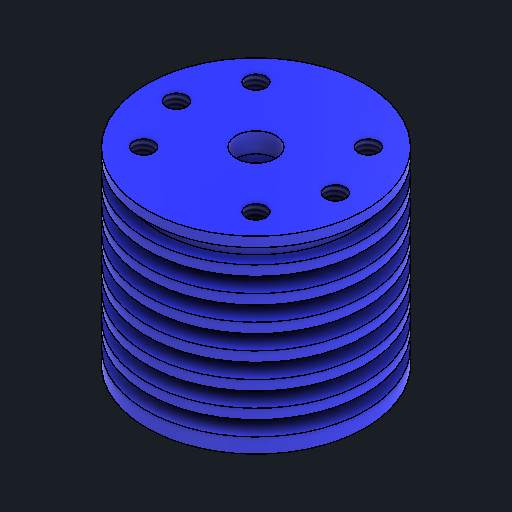
# Autodesk Inventor part: Radiator
Saved by Autodesk Inventor 2026.1 (Build 301233020, 233B)
## iProperties
Created: 2025-11-13
Part Number: Radiator
Material: Aluminum 6061
Document SubType Name: Modeling
Designer: JoshuaEah
Density: 2.7 g/cm^3
Appearance: Blue - Wall Paint - Glossy
Author: JoshuaEah
Autodesk Inventor part; units mm, degrees
ref_plane "YZ Plane" through (0, 0, 0) normal (1, 0, 0) x (0, 1, 0)
ref_plane "XZ Plane" through (0, 0, 0) normal (0, 1, 0) x (-1, 0, 0)
ref_plane "XY Plane" through (0, 0, 0) normal (0, 0, 1) x (1, 0, 0)
sketch "Sketch1" plane through (0, 0, 0) normal (0, 1, 0) x (-1, 0, 0)
  circle A0 centre (0, 0) radius 11
  circle A1 centre (0, 0) radius 9.75
  circle A2 centre (0, 0) radius 2
  circle A3 centre (0, 0) radius 0.95
  circle A4 centre (0, 0) radius 4.5
  circle A5 centre (8, 0) radius 1.25
  circle A6 centre (5.6569, 5.6569) radius 1.25
  circle A7 centre (0, 8) radius 1.25
  circle A8 centre (-5.6569, 5.6569) radius 1.25
  circle A9 centre (-8, 0) radius 1.25
  circle A10 centre (-5.6569, -5.6569) radius 1.25
  circle A11 centre (0, -8) radius 1.25
  circle A12 centre (5.6569, -5.6569) radius 1.25
  circle A13 centre (0, 0) radius 6.5
  dimension "d0" = 22
  dimension "d3" = 19.5
  dimension "d8" = 4
  dimension "d9" = 1.9
  dimension "d10" = 9
  dimension "d13" = 2.5
  dimension "d14" = 8
  dimension "d17" = 360
  dimension "d26" = 13
  constraints: 14 centre point, 6 coincident, 1 horizontal alignment, 17 other
  measures "d0" diameter of A0
  measures "d3" diameter of A1
  measures "d8" diameter of A2
  measures "d9" diameter of A3
  measures "d10" diameter of A4
  measures "d13" diameter of A5
  measures "d14" distance of point (0, 0) A5.centre
  measures "d26" diameter of A13
extrude "Extrusion1" add sketch "Sketch1" against normal blind 1 contours A0 | A1 | A2 | A3 | A4 | A5 | A6 | A7 | A8 | A9 | A10 | A11 | A12 | A13
extrude "Extrusion2" add sketch "Sketch1" against normal blind 1.5 from surface at -1 contours A1 | A2 | A3 | A4 | A5 | A6 | A7 | A8 | A9 | A10 | A11 | A12 | A13
extrude "Extrusion3" add sketch "Sketch1" against normal blind 1 from surface at -2.5 contours A0 | A1 | A2 | A3 | A4 | A5 | A6 | A7 | A8 | A9 | A10 | A11 | A12 | A13
extrude "Extrusion4" add sketch "Sketch1" against normal blind 1.5 from surface at -3.5 contours A2 | A3 | A4
extrude "Extrusion5" add sketch "Sketch1" against normal blind 1 from surface at -5 contours A0 | A1 | A2 | A3 | A4 | A5 | A6 | A7 | A8 | A9 | A10 | A11 | A12 | A13
pattern_linear "Rectangular Pattern1" count 5 spacing 2.5 along (0, -1, 0) of "Extrusion4", "Extrusion5"
extrude "Extrusion6" add sketch "Sketch1" against normal blind 1.5 from surface at -16 contours A2 | A3 | A4 | A13
extrude "Extrusion7" add sketch "Sketch1" against normal blind 1.5 from surface at -17.5 contours A0 | A1 | A2 | A3 | A4 | A5 | A6 | A7 | A8 | A9 | A10 | A11 | A12 | A13
hole "Hole1" at (0, 0, 0) direction (0, -1, 0) diameter 4 depth 2
hole "Hole2" at (0, 0, 0) direction (0, -1, 0) diameter 1.9 end through all
hole "Hole3" at (-5.6569, 0, -5.6569) at (-8, 0, 0) at (-5.6569, 0, 5.6569) at (5.6569, 0, 5.6569) at (8, 0, 0) at (5.6569, 0, -5.6569) direction (0, -1, 0) diameter 2.013 depth 3.5 thread size "M2.5x0.45" class "6H" standard "ANSI Metric M Profile"
sketch "Sketch2" plane through (0, -19, 0) normal (0, -1, 0) x (1, 0, 0)
  circle A0 centre (-5.1, 0) radius 1.25
  circle A1 centre (0, 0) radius 11 projected
  line L0 (0, 11) -> (0, -11)
  circle A2 centre (5.1, 0) radius 1.25
  dimension "d52" = 2.5
  dimension "d68" = 10.2
  constraints: 2 centre point, 2 end point, 2 point on circle, 1 horizontal alignment, 1 midpoint, 1 symmetric about line, 1 vertical, 1 other
  measures "d52" diameter of A0
  measures "d68" diameter of A0.centre L0
hole "Hole4" at (-5.1, -19, 0) at (5.1, -19, 0) direction (0, 1, 0) diameter 1.221 depth 4 thread size "M1.6x0.35" class "6H" standard "ANSI Metric M Profile"
hole "Hole5" at (0, -19, 0) direction (0, 1, 0) diameter 4 depth 15.5
equation "\"d31\" = d8"
equation "\"d38\" = d9"
body "Solid1"
